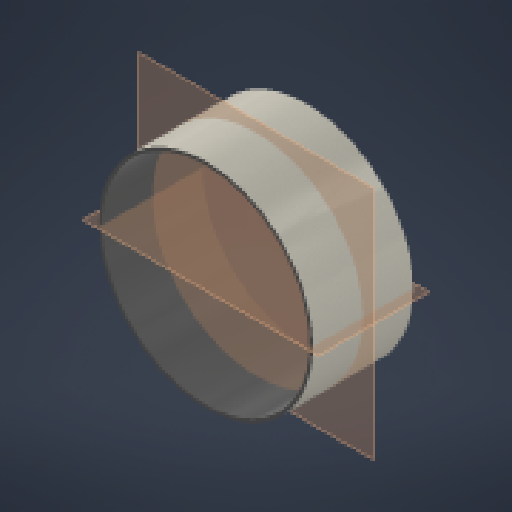
# Autodesk Inventor part: Rouleau
Saved by Autodesk Inventor 2026.2 (Build 302298010, 298A)
## iProperties
Created: 2026-03-28
Part Number: Rouleau
Material: Générique
Document SubType Name: Modeling
Designer: romai
Density: 1 g/cm^3
Appearance: Par défaut
Author: romai
Autodesk Inventor part; units mm, degrees
ref_plane "YZ Plane" through (0, 0, 0) normal (1, 0, 0) x (0, 1, 0)
ref_plane "XY Plane" through (0, 0, 0) normal (0, 0, 1) x (1, 0, 0)
sketch "Esquisse1" plane through (0, 0, 0) normal (0, 0, 1) x (1, 0, 0)
  circle A0 centre (0, 0) radius 77.5
  circle A1 centre (0, 0) radius 80
  dimension "d0" = 155
  dimension "d1" = 160
  constraints: 2 centre point, 2 coincident
  measures "d0" diameter of A0
  measures "d1" diameter of A1
extrude "Extrusion1" add sketch "Esquisse1" against normal blind 70
ref_plane "Plan de construction1" through (0, 0, -35) normal (0, 0, 1) x (1, 0, 0)
